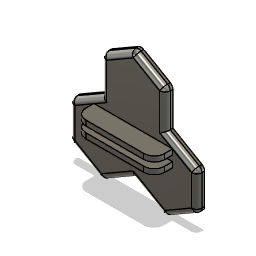
Hex Base Large (Autodesk Fusion 360 design; units mm, degrees)
Autodesk Fusion 360 part; units mm, degrees
sketch "Sketch1" plane through (0, 0, 0) normal (0, 0, 1) x (1, 0, 0)
  line L0 (0, 0) -> (-12.1, 6.9859) construction
  line L1 (0, 0) -> (0, -13.9719) construction
  line L2 (0, 0) -> (12.1, 6.9859) construction
  line L3 (12.1, -20.9578) -> (24.2, -13.9719)
  line L4 (24.2, -13.9719) -> (24.2, 0)
  line L5 (24.2, 0) -> (12.1, 6.9859)
  line L6 (12.1, 6.9859) -> (0, 0)
  line L7 (0, 0) -> (0, -13.9719)
  line L8 (0, -13.9719) -> (12.1, -20.9578)
  line L9 (12.1, 6.9859) -> (12.1, 20.9578)
  line L10 (12.1, 20.9578) -> (0, 27.9438)
  line L11 (0, 27.9438) -> (-12.1, 20.9578)
  line L12 (-12.1, 20.9578) -> (-12.1, 6.9859)
  line L13 (-12.1, 6.9859) -> (0, 0)
  line L14 (0, 0) -> (12.1, 6.9859) construction
  line L15 (0, -13.9719) -> (0, 0) construction
  line L16 (0, 0) -> (-12.1, 6.9859)
  line L17 (-12.1, 6.9859) -> (-24.2, 0)
  line L18 (-24.2, 0) -> (-24.2, -13.9719)
  line L19 (-24.2, -13.9719) -> (-12.1, -20.9578)
  line L20 (-12.1, -20.9578) -> (0, -13.9719)
  point P0 (12.1, -6.9859)
  point P1 (0, 13.9719)
  point P2 (-12.1, -6.9859)
  dimension "d3" = 120
  dimension "d4" = 120
  dimension "d5" = 12.1
  dimension "d6" = 12.1
  dimension "d7" = 12.1
  constraint coincident L0.start L1.start
  constraint collinear L0 L16
  constraint collinear L1 L15
  constraint collinear L1 L7
  constraint collinear L2 L6
  constraint collinear L0 L13
  constraint collinear L2 L14
  constraint coincident L0.end L12.end
  constraint coincident L2.end L5.end
  constraint coincident L1.end L7.end
  constraint vertical L1
  measures "d3" angle of L1 L2
  measures "d4" angle of L0 L2
  measures "d5" distance of P0 L8
  measures "d6" distance of P1 L14
  measures "d7" distance of P2 L20
extrude "Extrude1" add sketch "Sketch1" along normal blind 3
sketch "Sketch2" plane through (0, 0, 3) normal (0, 0, 1) x (1, 0, 0)
  line L0 (-12.1, -20.9578) -> (0, -13.9719)
  line L1 (0, -13.9719) -> (12.1, -20.9578)
  line L2 (12.1, -20.9578) -> (24.2, -13.9719)
  line L3 (24.2, -13.9719) -> (24.2, 0)
  line L4 (24.2, 0) -> (12.1, 6.9859)
  line L5 (12.1, 6.9859) -> (12.1, 20.9578)
  line L6 (12.1, 20.9578) -> (0, 27.9438)
  line L7 (0, 27.9438) -> (-12.1, 20.9578)
  line L8 (-12.1, 20.9578) -> (-12.1, 6.9859)
  line L9 (-12.1, 6.9859) -> (-24.2, 0)
  line L10 (-24.2, 0) -> (-24.2, -13.9719)
  line L11 (-24.2, -13.9719) -> (-12.1, -20.9578)
  line L12 (15, 1.1) -> (-15, 1.1)
  line L13 (-15, 1.1) -> (-15, 3.1)
  line L14 (-15, 3.1) -> (15, 3.1)
  line L15 (15, 3.1) -> (15, 1.1)
  line L16 (15, -1.1) -> (-15, -1.1)
  line L17 (-15, -1.1) -> (-15, -3.1)
  line L18 (-15, -3.1) -> (15, -3.1)
  line L19 (15, -3.1) -> (15, -1.1)
  line L20 (24.2, -13.9719) -> (-12.1, 6.9859) construction
  line L21 (-24.2, -13.9719) -> (12.1, 6.9859) construction
  line L22 (0, 27.9438) -> (0, -13.9719) construction
  line L23 (24.2, -13.9719) -> (24.2, 0)
  line L24 (24.2, 0) -> (-24.2, 0) construction
  dimension "d10" = 30
  dimension "d11" = 2
  dimension "d16" = 2.2
  constraint perpendicular L12 L13
  constraint parallel L12 L14
  constraint parallel L13 L15
  constraint perpendicular L16 L17
  constraint parallel L16 L18
  constraint parallel L17 L19
  constraint equal L15 L19
  constraint equal L12 L16
  constraint parallel L12 L16
  constraint collinear L15 L19
  constraint coincident L2.end L3.start
  constraint coincident L8.end L9.start
  constraint coincident L10.end L11.start
  constraint coincident L4.end L5.start
  constraint coincident L6.end L7.start
  constraint coincident L0.end L1.start
  constraint horizontal L14
  constraint coincident L3.end L4.start
  constraint coincident L9.end L10.start
  constraint symmetric L12 L16 L24
  constraint symmetric L13 L15 L22
  measures "d10" distance of L12.start L12.end
  measures "d11" distance of L12.start L14.end
  measures "d16" distance of L12 L16
extrude "Extrude2" add sketch "Sketch2" along normal blind 7 contours L12 L13 L14 L15 | L16 L17 L18 L19
sketch "Sketch3" plane through (0, 0, 0) normal (0, 0, -1) x (-1, 0, 0)
  line L0 (0, -13.9719) -> (12.1, -20.9578)
  line L1 (12.1, -20.9578) -> (24.2, -13.9719)
  line L2 (24.2, -13.9719) -> (24.2, 0)
  line L3 (24.2, 0) -> (12.1, 6.9859)
  line L4 (12.1, 6.9859) -> (12.1, 20.9578)
  line L5 (12.1, 20.9578) -> (0, 27.9438)
  line L6 (0, 27.9438) -> (-12.1, 20.9578)
  line L7 (-12.1, 20.9578) -> (-12.1, 6.9859)
  line L8 (-12.1, 6.9859) -> (-24.2, 0)
  line L9 (-24.2, 0) -> (-24.2, -13.9719)
  line L10 (-24.2, -13.9719) -> (-12.1, -20.9578)
  line L11 (-12.1, -20.9578) -> (0, -13.9719)
  line L12 (-15, 1.05) -> (15, 1.05)
  line L13 (15, 1.05) -> (15, -1.05)
  line L14 (15, -1.05) -> (-15, -1.05)
  line L15 (-15, -1.05) -> (-15, 1.05)
  line L16 (-15, 0) -> (15, 0) construction
  line L17 (0, -1.05) -> (0, 1.05) construction
  dimension "d19" = 30
  dimension "d20" = 2.1
  constraint horizontal L12
  constraint vertical L13
  constraint horizontal L14
  constraint vertical L15
  constraint midpoint L15 L16.start
  constraint midpoint L13 L16.end
  constraint midpoint L14 L17.start
  constraint midpoint L12 L17.end
  constraint midpoint L16 origin
  measures "d19" distance of L12.start L12.end
  measures "d20" distance of L12.start L14.end
extrude "Extrude3" cut sketch "Sketch3" against normal blind 2 contours L12 L13 L14 L15
fillet "Fillet1" radius 4 4 edges at (15, 2.1, 10) (15, -2.1, 10) (-15, 2.1, 10) (-15, -2.1, 10)
fillet "Fillet2" radius 2 9 edges at (-12.1, -20.9578, 1.5) (12.1, -20.9578, 1.5) (24.2, -13.9719, 1.5) (24.2, 0, 1.5) (12.1, 20.9578, 1.5) (0, 27.9438, 1.5) (-12.1, 20.9578, 1.5) (-24.2, 0, 1.5) (-24.2, -13.9719, 1.5)
fillet "Fillet3" radius 0.5 4 edges at (0, -1.05, 0) (0, 1.05, 0) (-15, 0, 0) (15, 0, 0)
fillet "Fillet5" radius 2 21 edges at (12.1, 13.3945, 3) (11.8321, 20.8031, 3) (6.05, 24.4508, 3) (0, 27.6344, 3) (-6.05, 24.4508, 3) (-11.8321, 20.8031, 3) (-12.1, 13.3945, 3) (5.55, -17.1762, 3) (12.1, -20.6484, 3) (18.15, -17.4648, 3) (23.9321, -13.8172, 3) (24.2, -6.9859, 3) (23.9321, -0.1547, 3) (17.65, 3.7816, 3) (-17.65, 3.7816, 3) (-23.9321, -0.1547, 3) (-24.2, -6.9859, 3) (-23.9321, -13.8172, 3) (-18.15, -17.4648, 3) (-12.1, -20.6484, 3) (-5.55, -17.1762, 3)
named bodies: "Hex Base Large"
